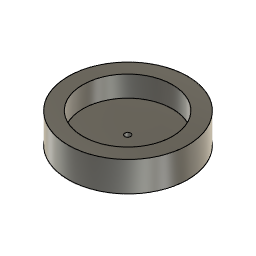
theAlarmClock_3D (Autodesk Fusion 360 archive; units mm, degrees)
design "rengasv3"
Autodesk Fusion 360 part; units mm, degrees
sketch "Sketch1" plane through (0, 0, 0) normal (0, 0, 1) x (1, 0, 0)
  circle A0 centre (0, 0) radius 20
  constraint coincident A0.centre origin
extrude "Extrude1" add sketch "Sketch1" along normal blind 10
hole "Hole1" at (-0.1278, 0, 10) direction (0, 0, -1) diameter 30 depth 7 tip angle 180
hole "Hole2" at (-0.0621, -0.0347, 0) direction (0, 0, 1) diameter 2 depth 7 tip angle 180
